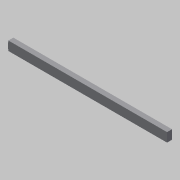
# Autodesk Inventor part: pin_interconnect
Saved by Autodesk Inventor 2019.3 (Build 233278000, 278)
## iProperties
Created: 2019-02-28
Part Number: pin_interconnect
Material: Generic
Document SubType Name: Modeling
Designer: Varga Daniel
Density: 1 g/cm^3
Appearance: Default
Author: Varga Daniel
Autodesk Inventor part; units mm, degrees
ref_plane "YZ Plane" through (0, 0, 0) normal (1, 0, 0) x (0, 1, 0)
ref_plane "XZ Plane" through (0, 0, 0) normal (0, 1, 0) x (-1, 0, 0)
ref_plane "XY Plane" through (0, 0, 0) normal (0, 0, 1) x (1, 0, 0)
sketch "Sketch1" plane through (0, 0, 0) normal (0, 0, 1) x (1, 0, 0)
  line L0 (-2.2452, 0) -> (5.8622, 0) projected
  line L1 (-1, 1) -> (1, 1)
  line L2 (1, 1) -> (1, -1)
  line L3 (1, -1) -> (-1, -1)
  line L4 (-1, -1) -> (-1, 1)
  line L5 (-1, 1) -> (1, -1) construction
  line L6 (1, 1) -> (-1, -1) construction
  arc A0 (-1, 1) -> (-1, -1) centre (4.704, 0) ccw
  point P0 (0, 0)
  dimension "d11" = 2
  dimension "d12" = 2
  constraints: 12 end point, 2 midpoint, 2 parallel, 2 point on circle, 1 centre point, 1 horizontal, 1 perpendicular, 1 point on line
  measures "d11" distance of L2.end L3.end
  measures "d12" distance of L1.end L2.end
extrude "Extrusion2" add sketch "Sketch1" along normal blind 1.1
move faces "Move1" translate (33, 0, 0) faces at (1, 0.3333, 0.3667)
body "Solid2"
